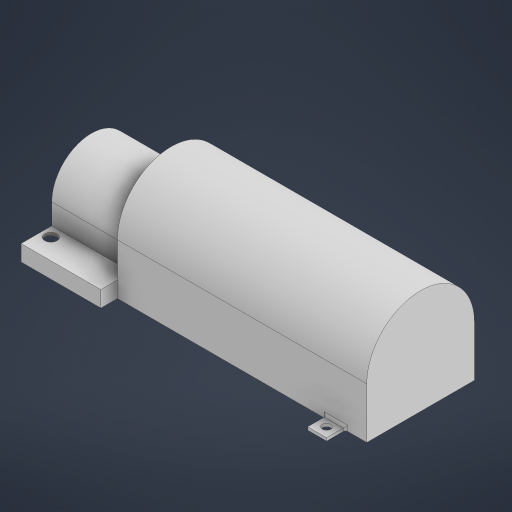
# Autodesk Inventor part: carcasa_motores
Saved by Autodesk Inventor 2023.1 (Build 271208000, 208)
## iProperties
Created: 2022-11-15
Part Number: carcasa_motores
Material: Generic
Document SubType Name: Modeling
Designer: amtat
Density: 1 g/cm^3
Appearance: Default
Author: amtat
Autodesk Inventor part; units mm, degrees
ref_plane "YZ Plane" through (0, 0, 0) normal (1, 0, 0) x (0, 1, 0)
ref_plane "XZ Plane" through (0, 0, 0) normal (0, 1, 0) x (-1, 0, 0)
ref_plane "XY Plane" through (0, 0, 0) normal (0, 0, 1) x (1, 0, 0)
sketch "Sketch1" plane through (0, 0, 0) normal (1, 0, 0) x (0, 1, 0)
  arc A0 (0, -15.5) -> (0, 15.5) centre (0, 0) ccw
  line L0 (0, -15.5) -> (-10, -15.5)
  line L1 (0, -15.5) -> (0, -16.75)
  arc A1 (0, -16.75) -> (0, 16.75) centre (0, 0) ccw
  line L2 (0, -16.75) -> (-10, -16.75)
  line L3 (-10, -15.5) -> (-10, -27.5)
  line L4 (-10, -16.75) -> (-8.75, -16.75)
  line L5 (-8.75, -27.5) -> (-8.75, -28.75)
  line L6 (-15.5, 0) -> (-15.5, -28.75)
  line L7 (-8.75, -27.5) -> (-8.75, -16.75)
  line L8 (0, 0) -> (-6.7436, 0)
  line L9 (0, 15.5) -> (-10, 15.5)
  line L10 (0, 16.75) -> (-8.75, 16.75)
  line L11 (-10, 15.5) -> (-10, 27.5)
  line L12 (-8.75, 27.5) -> (-8.75, 28.75)
  line L13 (-15.5, 0) -> (-15.5, 28.75)
  line L14 (-8.75, 27.5) -> (-8.75, 16.75)
  line L15 (-10, -27.5) -> (-10, -28.5)
  line L16 (-10, -28.5) -> (-15.5, -28.5)
  line L17 (-15.5, -28.5) -> (-15.5, -29.75)
  line L18 (-15.5, -29.75) -> (-8.75, -29.75)
  line L19 (-8.75, -29.75) -> (-8.75, -28.75)
  line L20 (-8.75, 27.5) -> (-8.75, 28.75)
  line L21 (-10, 27.5) -> (-10, 28.5)
  line L22 (-10, 28.5) -> (-15.5, 28.5)
  line L23 (-15.5, 28.5) -> (-15.5, 29.75)
  line L24 (-15.5, 29.75) -> (-8.75, 29.75)
  line L25 (-8.75, 29.75) -> (-8.75, 28.75)
  point P0 (-10, 16.75)
  dimension "d0" = 31
  dimension "d1" = 10
  dimension "d2" = 1.25
  dimension "d3" = 12
  dimension "d4" = 1.25
  dimension "d5" = 1.25
  dimension "d6" = 1
  dimension "d7" = 1.25
  constraints: 52 end point, 13 symmetric about line, 5 vertical, 4 point on circle, 3 horizontal, 3 perpendicular, 2 centre point, 2 coincident, 2 point on line, 2 tangent
  measures "d0" diameter of A0
  measures "d1" distance of L0.start L0.end
  measures "d2" distance of L0.start L1.end
  measures "d3" distance of L0.end L3.end
  measures "d4" distance of L2.end L4.end
  measures "d5" distance of L5.start L5.end
  measures "d6" distance of L3.end L15.end
  measures "d7" distance of L16.end L17.end
extrude "Extrusion1" add sketch "Sketch1" along normal blind 35 contours L1 L2 L3 L0 | A0 L9 L11 L21 L22 L13 L23 L24 L25 L12 L14 L10 A1 L1 | L2 L7 L5 L19 L18 L17 L6 L16 L15 L3
sketch "Sketch2" plane through (35, 0, 0) normal (1, 0, 0) x (0, 0, -1)
  line L0 (29.75, -8.75) -> (16.75, -8.75) projected
  line L1 (16.75, -8.75) -> (16.75, 0) projected
  arc A0 (16.75, 0) -> (-16.75, 0) centre (0, 0) ccw projected
  line L2 (-16.75, 0) -> (-16.75, -8.75) projected
  line L3 (-16.75, -8.75) -> (-29.75, -8.75) projected
  line L4 (-29.75, -8.75) -> (-29.75, -15.5) projected
  line L5 (-29.75, -15.5) -> (-28.5, -15.5) projected
  line L6 (-28.5, -15.5) -> (-28.5, -10) projected
  line L7 (-28.5, -10) -> (-15.5, -10) projected
  line L8 (-15.5, -10) -> (-15.5, 0) projected
  arc A1 (15.5, 0) -> (-15.5, 0) centre (0, 0) ccw projected
  line L9 (15.5, 0) -> (15.5, -10) projected
  line L10 (15.5, -10) -> (28.5, -10) projected
  line L11 (28.5, -10) -> (28.5, -15.5) projected
  line L12 (28.5, -15.5) -> (29.75, -15.5) projected
  line L13 (29.75, -15.5) -> (29.75, -8.75) projected
  line L14 (-28.5, -15.5) -> (-28.5, -10) projected
  line L15 (-28.5, -15.5) -> (0, -15.5)
  line L16 (0, -15.5) -> (0, 27.5)
  line L17 (0, 27.5) -> (0, 6)
  line L18 (21.5, 6) -> (21.5, -15.5)
  line L19 (21.5, -15.5) -> (22.75, -15.5)
  line L20 (22.75, -15.5) -> (22.75, 6)
  line L21 (-21.5, 6) -> (-21.5, -15.5)
  line L22 (-21.5, -15.5) -> (-22.75, -15.5)
  line L23 (-22.75, -15.5) -> (-22.75, 6)
  arc A2 (22.75, 6) -> (-22.75, 6) centre (0, 6) ccw
  arc A3 (-17.3205, -8.75) -> (-16.1729, -10) centre (0, 6) ccw
  arc A4 (16.1729, -10) -> (17.3205, -8.75) centre (0, 6) ccw
  arc A5 (-16.75, -7.4792) -> (-15.5, -8.8997) centre (0, 6) ccw
  arc A6 (15.5, -8.8997) -> (16.75, -7.4792) centre (0, 6) ccw
  arc A7 (21.5, 6) -> (-21.5, 6) centre (0, 6) ccw
  dimension "d10" = 43
  dimension "d11" = 21.5
  dimension "d12" = 1.25
  constraints: 18 end point, 13 point on circle, 7 point on line, 6 centre point, 4 symmetric about line, 3 perpendicular, 2 coincident, 1 horizontal, 1 midpoint, 1 tangent, 1 vertical
  measures "d10" distance of L15.end L16.end
  measures "d11" distance of L16.end L17.end
  measures "d12" distance of L18.end L19.end
extrude "Extrusion2" add sketch "Sketch2" along normal blind 103 contours L18 A7 L21 L3 L23 A2 L20 L0 | L0 L20 L10 L18 | L10 L20 L19 L18 | L3 L21 L7 L23 | L7 L21 L15 L23
sketch "Sketch3" plane through (35, 0, 0) normal (-1, 0, 0) x (0, 0, 1)
  line L0 (-22.75, -8.75) -> (-21.5, -8.75) projected
  line L1 (-21.5, 6) -> (-21.5, -8.75) projected
  arc A0 (21.5, 6) -> (-21.5, 6) centre (0, 6) ccw projected
  line L2 (21.5, -8.75) -> (21.5, 6) projected
  line L3 (21.5, -8.75) -> (22.75, -8.75) projected
  line L4 (22.75, 6) -> (22.75, -8.75) projected
  arc A1 (22.75, 6) -> (-22.75, 6) centre (0, 6) ccw projected
  line L5 (-22.75, -8.75) -> (-22.75, 6) projected
  line L6 (-29.75, -8.75) -> (-16.75, -8.75) projected
  line L7 (-29.75, -15.5) -> (-29.75, -8.75) projected
  line L8 (-28.5, -15.5) -> (-29.75, -15.5) projected
  line L9 (-28.5, -10) -> (-28.5, -15.5) projected
  line L10 (-15.5, -10) -> (-28.5, -10) projected
  line L11 (-15.5, 0) -> (-15.5, -10) projected
  arc A2 (15.5, 0) -> (-15.5, 0) centre (0, 0) ccw projected
  line L12 (15.5, -10) -> (15.5, 0) projected
  line L13 (28.5, -10) -> (15.5, -10) projected
  line L14 (28.5, -15.5) -> (28.5, -10) projected
  line L15 (29.75, -15.5) -> (28.5, -15.5) projected
  line L16 (29.75, -8.75) -> (29.75, -15.5) projected
  line L17 (16.75, -8.75) -> (29.75, -8.75) projected
  line L18 (16.75, 0) -> (16.75, -8.75) projected
  arc A3 (16.75, 0) -> (-16.75, 0) centre (0, 0) ccw projected
  line L19 (-16.75, -8.75) -> (-16.75, 0) projected
extrude "Extrusion3" add sketch "Sketch3" along normal blind 1.25 contours L5 A1 L4 L3 L2 A0 L1 L0 | L1 A0 L2 L17 L18 A3 L19 L6
sketch "Sketch4" plane through (0, -8.75, 29.75) normal (0, 1, 0) x (1, 0, 0)
  line L0 (33.75, 7) -> (33.75, 13) projected
  line L1 (0, 13) -> (33.75, 13) projected
  line L2 (0, 13) -> (0, 0) projected
  line L3 (0, 0) -> (35, 0) projected
  line L4 (35, 7) -> (35, 0) projected
  line L5 (35, 7) -> (33.75, 7) projected
  line L6 (33.75, 46.5) -> (33.75, 52.5) projected
  line L7 (33.75, 52.5) -> (35, 52.5) projected
  line L8 (35, 59.5) -> (35, 52.5) projected
  line L9 (0, 59.5) -> (35, 59.5) projected
  line L10 (0, 59.5) -> (0, 46.5) projected
  line L11 (0, 46.5) -> (33.75, 46.5) projected
  line L12 (33.75, 7) -> (33.75, 0)
  line L13 (0, 0) -> (35, 0) projected
  line L14 (33.75, 52.5) -> (33.75, 59.5)
  line L15 (0, 59.5) -> (35, 59.5) projected
  point P0 (0, 29.75)
  constraints: 4 end point, 3 point on line, 1 vertical
extrude "Extrusion4" cut sketch "Sketch4" against normal through all contours L5 L4 L3 L12 | L14 L9 L8 L7
sketch "Sketch5" plane through (35, 0, 0) normal (-1, 0, 0) x (0, 0, 1)
  line L0 (-21.5, -10) -> (-22.75, -10) projected
  line L1 (-22.75, -15.5) -> (-22.75, -10) projected
  line L2 (-21.5, -15.5) -> (-22.75, -15.5) projected
  line L3 (-21.5, -10) -> (-21.5, -15.5) projected
  line L4 (22.75, -10) -> (21.5, -10) projected
  line L5 (21.5, -15.5) -> (21.5, -10) projected
  line L6 (22.75, -15.5) -> (21.5, -15.5) projected
  line L7 (22.75, -10) -> (22.75, -15.5) projected
  point P0 (0, 0)
extrude "Extrusion5" add sketch "Sketch5" along normal blind 2.5
sketch "Sketch6" plane through (138, -15.5, 22.75) normal (0, 0, 1) x (1, 0, 0)
  line L0 (-104.25, 0) -> (-104.25, 6.75) projected
  line L1 (-138, 6.75) -> (-104.25, 6.75) projected
  line L2 (-138, 6.75) -> (-138, 0) projected
  line L3 (-138, 0) -> (-104.25, 0) projected
  line L4 (-105.5, 0) -> (-105.5, 5.5) projected
  line L5 (-105.5, 5.5) -> (-104.25, 5.5) projected
  point P0 (-138, 15.5)
extrude "Extrusion6" add sketch "Sketch6" along normal blind 7 contours L3 L4 L5 L0
sketch "Sketch7" plane through (138, -15.5, -22.75) normal (0, 0, -1) x (-1, 0, 0)
  line L0 (104.25, 6.75) -> (104.25, 0) projected
  line L1 (105.5, 5.5) -> (105.5, 0) projected
  line L2 (103, 5.5) -> (105.5, 5.5) projected
  line L3 (105.5, 0) -> (0, 0) projected
  point P0 (138, 15.5)
  point P1 (104.25, 5.5)
extrude "Extrusion7" add sketch "Sketch7" along normal blind 7
sketch "Sketch8" plane through (138, 0, 0) normal (1, 0, 0) x (0, 0, -1)
  line L0 (-22.75, 6) -> (-22.75, -15.5) projected
  line L1 (-22.75, -15.5) -> (-21.5, -15.5) projected
  line L2 (-21.5, -15.5) -> (-21.5, 6) projected
  arc A0 (21.5, 6) -> (-21.5, 6) centre (0, 6) ccw projected
  line L3 (21.5, 6) -> (21.5, -15.5) projected
  line L4 (21.5, -15.5) -> (22.75, -15.5) projected
  line L5 (22.75, -15.5) -> (22.75, 6) projected
  arc A1 (22.75, 6) -> (-22.75, 6) centre (0, 6) ccw projected
  line L6 (-22.75, -15.5) -> (22.75, -15.5)
  line L7 (-21.5, -15.5) -> (-28.5, -15.5) projected
  point P0 (0, 0)
  constraints: 2 end point, 1 collinear
extrude "Extrusion8" add sketch "Sketch8" along normal blind 1.25
sketch "Sketch9" plane through (33.75, -8.75, 22.75) normal (0, 0, 1) x (1, 0, 0)
  line L0 (0, 0) -> (0, -6.75) projected
  line L1 (0, -6.75) -> (105.5, -6.75) projected
  line L2 (105.5, 14.75) -> (105.5, -6.75) projected
  line L3 (105.5, 14.75) -> (0, 14.75) projected
  line L4 (0, 0) -> (0, 14.75) projected
  line L5 (105.5, -6.75) -> (96.5, -6.75)
  line L6 (-1.25, -6.75) -> (104.25, -6.75) projected
  line L7 (96.5, -6.75) -> (96.5, -5.5)
  line L8 (96.5, -5.5) -> (88.5, -5.5)
  line L9 (88.5, -5.5) -> (88.5, -6.75)
  point P0 (-33.75, 8.75)
  dimension "d27" = 9
  dimension "d28" = 1.25
  dimension "d29" = 8
  constraints: 8 end point, 2 perpendicular, 2 point on line, 1 horizontal
  measures "d27" distance of L1.end L5.end
  measures "d28" distance of L5.end L7.end
  measures "d29" distance of L7.end L8.end
extrude "Extrusion9" add sketch "Sketch9" along normal blind 8 contours L9 L8 L7 L1
sketch "Sketch10" plane through (33.75, -8.75, -22.75) normal (0, 0, -1) x (-1, 0, 0)
  line L0 (-88.5, -6.75) -> (-96.5, -6.75) projected
  line L1 (-88.5, -5.5) -> (-88.5, -6.75) projected
  line L2 (-88.5, -6.75) -> (-96.5, -6.75) projected
  line L3 (-96.5, -6.75) -> (-96.5, -5.5) projected
  line L4 (-96.5, -5.5) -> (-88.5, -5.5) projected
  point P0 (33.75, 8.75)
extrude "Extrusion10" add sketch "Sketch10" along normal blind 8
sketch "Sketch11" plane through (122.25, -14.25, -22.75) normal (0, 1, 0) x (1, 0, 0)
  line L0 (8, 0) -> (0, 0) projected
  line L1 (8, 0) -> (8, 8) projected
  line L2 (0, 8) -> (8, 8) projected
  line L3 (0, 0) -> (0, 8) projected
  line L4 (0, -45.5) -> (8, -45.5) projected
  line L5 (0, -45.5) -> (0, -53.5) projected
  line L6 (8, -53.5) -> (0, -53.5) projected
  line L7 (8, -45.5) -> (8, -53.5) projected
  line L8 (0, -45.5) -> (0, -53.5) projected
  line L9 (0, -53.5) -> (4, -53.5)
  line L10 (0, -53.5) -> (8, -53.5) projected
  line L11 (4, -53.5) -> (4, -49.5)
  circle A0 centre (4, -49.5) radius 1.8
  line L12 (0, 8) -> (8, 8) projected
  line L13 (8, 8) -> (4, 8)
  line L14 (8, 8) -> (12, 8) construction
  line L15 (4, 8) -> (4, 4)
  line L16 (0, 0) -> (0, 8) projected
  circle A1 centre (4, 4) radius 1.8
  point P0 (-122.25, -22.75)
  dimension "d34" = 4
  dimension "d35" = 3.6
  dimension "d36" = 4
  dimension "d37" = 180
  dimension "d38" = 3.6
  constraints: 10 end point, 2 centre point, 2 coincident, 2 collinear, 1 horizontal, 1 midpoint, 1 parallel, 1 perpendicular
  measures "d34" distance of L5.end L9.end
  measures "d35" diameter of A0
  measures "d36" distance of L1.end L13.end
  measures "d37" angle of L13 L14
  measures "d38" diameter of A1
extrude "Extrusion11" cut sketch "Sketch11" against normal blind 8 contours A1 | A0
fillet "Fillet1" radius 1 6 edges at (130.25, -14.875, 22.75) (126.25, -14.25, 22.75) (122.25, -14.875, 22.75) (130.25, -14.875, -22.75) (126.25, -14.25, -22.75) (122.25, -14.875, -22.75)
fillet "Fillet2" radius 2 3 edges at (33.75, -4.375, -16.75) (33.75, -4.375, 16.75) (33.75, 16.75, 0)
sketch "Sketch12" plane through (0, -8.75, -16.75) normal (0, 1, 0) x (1, 0, 0)
  arc A0 (31.75, 0) -> (33.75, 2) centre (31.75, 2) ccw projected
  line L0 (33.75, 2) -> (33.75, 6) projected
  line L1 (33.75, 6) -> (33.75, 13) projected
  line L2 (0, 13) -> (33.75, 13) projected
  line L3 (0, 13) -> (0, 0) projected
  line L4 (0, 0) -> (31.75, 0) projected
  arc A1 (33.75, -35.5) -> (31.75, -33.5) centre (31.75, -35.5) ccw projected
  line L5 (0, -33.5) -> (31.75, -33.5) projected
  line L6 (0, -33.5) -> (0, -46.5) projected
  line L7 (0, -46.5) -> (33.75, -46.5) projected
  line L8 (33.75, -46.5) -> (33.75, -39.5) projected
  line L9 (33.75, -39.5) -> (33.75, -35.5) projected
  line L10 (0, 13) -> (-2.5, 13)
  line L11 (-2.5, 13) -> (4, 13)
  line L12 (0, 13) -> (33.75, 13) projected
  line L13 (4, 13) -> (4, 8.75)
  line L14 (4, 8.75) -> (4, 4.4)
  circle A2 centre (4, 4.4) radius 2.55
  line L15 (0, 0) -> (0, -16.75)
  line L16 (0, -16.75) -> (16.875, -16.75)
  circle A3 centre (4, -37.9) radius 2.55
  dimension "d43" = 2.5
  dimension "d44" = 6.5
  dimension "d45" = 4.25
  dimension "d46" = 4.35
  dimension "d47" = 5.1
  constraints: 12 end point, 2 centre point, 2 horizontal, 2 vertical, 1 coincident, 1 perpendicular, 1 point on line, 1 symmetric about line, 1 other
  measures "d43" distance of L2.start L10.end
  measures "d44" distance of L10.end L11.end
  measures "d45" distance of L11.end L13.end
  measures "d46" distance of L13.end L14.end
  measures "d47" diameter of A2
extrude "Extrusion12" cut sketch "Sketch12" against normal blind 8 contours A2 | A3
body "Solid1"
